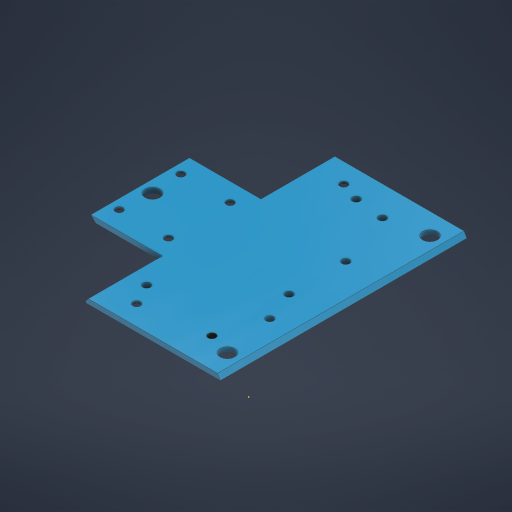
# Autodesk Inventor part: podstawa
Saved by Autodesk Inventor 2024 (Build 280153000, 153)
## iProperties
Created: 2024-05-21
Part Number: podstawa
Material: Steel
Document SubType Name: Modeling
Designer: Adam
Density: 7.85 g/cm^3
Appearance: Plate
Mass: 100.47 g
Surface Area: 136.936 cm^2
Volume: 12.7988 cm^3
Author: Adam
Autodesk Inventor part; units mm, degrees
ref_plane "YZ Plane" through (0, 0, 0) normal (1, 0, 0) x (0, 1, 0)
ref_plane "XZ Plane" through (0, 0, 0) normal (0, 1, 0) x (-1, 0, 0)
ref_plane "XY Plane" through (0, 0, 0) normal (0, 0, 1) x (1, 0, 0)
sketch "Sketch1" plane through (0, 0, 0) normal (0, 1, 0) x (-1, 0, 0)
  line L0 (0, 0) -> (0, -100)
  line L1 (0, -100) -> (66, -100)
  line L2 (66, -100) -> (66, -70)
  line L3 (66, -70) -> (94, -70)
  line L4 (94, -70) -> (94, -30)
  line L5 (94, -30) -> (66, -30)
  line L6 (66, -30) -> (66, 0)
  line L7 (66, 0) -> (0, 0)
  dimension "d0" = 100
  dimension "d2" = 30
  dimension "d4" = 40
  dimension "d7" = 66
  dimension "d27" = 94
  constraints: 16 end point, 4 perpendicular, 2 point on line, 1 parallel, 1 vertical
  measures "d0" distance of L0.start L0.end
  measures "d2" distance of L1.end L2.end
  measures "d4" distance of L3.end L4.end
  measures "d7" distance of L0.end L1.end
  measures "d27" distance between parallel lines of L0 L4
extrude "Extrusion1" add sketch "Sketch1" along normal blind 2
ref_plane "Work Plane1" through (-66, 0, -50) normal (0, 0, 1) x (1, 0, 0)
sketch "Sketch2" plane through (0, 0, 0) normal (0, -1, 0) x (1, 0, 0)
  point P0 (0, 0)
  point P1 (-69.9994, -37.5)
  point P2 (-90, -37.5)
  point P3 (-69.9994, -62.5)
  point P4 (-90, -62.5)
hole "Hole1" at (-90, 0, -37.5) at (-69.9994, 0, -37.5) at (-69.9994, 0, -62.5) at (-90, 0, -62.5) direction (0, 1, 0) diameter 3.1 end through all
chamfer "Chamfer1" distance 1.5 angle 45 4 edges at (-90, 0, -60.95) (-69.9994, 0, -60.95) (-69.9994, 0, -35.95) (-90, 0, -35.95) measured on face at (-69.9994, 0, -60.45) measured on face at (-90, 0, -60.45) measured on face at (-69.9994, 0, -35.45) measured on face at (-90, 0, -35.45)
chamfer "Chamfer2" distance 2 angle 45 1 edges at (-94, 0, -50)
sketch "Sketch3" plane through (-66, 0, -50) normal (0, 0, 1) x (1, 0, 0)
  line L0 (66, -6) -> (58, -6)
  line L1 (58, -6) -> (45.307, 15.985)
  line L2 (66, 0) -> (66, 2) projected
  line L3 (0, 0) -> (66, 0) projected
  line L4 (45.307, 15.985) -> (66, 15.985)
  line L5 (66, 15.985) -> (66, -6)
  line L6 (66, -6) -> (66, -6)
  point P0 (66, 1)
  dimension "d22" = 8
  dimension "d23" = 120
  dimension "d24" = 6
  constraints: 10 end point, 2 horizontal, 2 perpendicular, 2 point on line, 1 midpoint
  measures "d22" distance of L0.start L1.start
  measures "d23" angle of L0 L1
  measures "d24" distance between parallel lines of L3 L0
extrude "Extrusion2" cut sketch "Sketch3" along normal through all both and the other way through all
chamfer "Chamfer3" distance 1 distance2 1.2 2 edges at (-66, 2, -15) (-66, 2, -85) measured on face at (-65.5, 2, -85) measured on face at (-65.5, 2, -15)
sketch "Sketch4" plane through (0, 0, 0) normal (0, -1, 0) x (1, 0, 0)
  line L0 (-67.7565, -100) -> (-11.4641, -100)
  line L1 (-11.4641, -100) -> (-11.4641, 0)
  line L2 (-11.4641, 0) -> (-67.7565, 0)
  point P0 (0, 0)
  point P1 (-53.4039, -92)
  point P2 (-53.4039, -8)
  point P3 (-11.4641, 0)
  dimension "d31" = 8
  dimension "d32" = 41.9398
  dimension "d33" = 41.9398
  dimension "d34" = 8
  dimension "d35" = 100
  constraints: 6 end point, 2 perpendicular, 1 coincident
  measures "d31" distance from line of L2 point (-53.404, -8)
  measures "d32" distance from line of L1 point (-53.404, -8)
  measures "d33" distance from line of L1 point (-53.404, -92)
  measures "d34" distance from line of L0 point (-53.404, -92)
  measures "d35" distance between parallel lines of L0 L2
hole "Hole2" at (-53.4039, 0, -92) at (-53.4039, 0, -8) direction (0, 1, 0) diameter 3.1 end through all
chamfer "Chamfer4" distance 1.5 angle 45 2 edges at (-53.4039, 0, -90.45) (-53.4039, 0, -6.45) measured on face at (-53.4039, 0, -89.95) measured on face at (-53.4039, 0, -5.95)
sketch "Sketch6" plane through (0, 2, 0) normal (0, 1, 0) x (1, 0, 0)
  line L0 (-11.4641, 100) -> (-11.4641, 0) projected
  line L1 (-12.6188, 100) -> (-11.4641, 100) projected
  line L2 (-12.6188, 0) -> (-12.6188, 100) projected
  line L3 (-11.4641, 0) -> (-12.6188, 0) projected
  line L4 (-12.6188, 100) -> (-65, 100) projected
  line L5 (-65, 0) -> (-12.6188, 0) projected
  line L6 (-12.6715, 100) -> (-66, 100)
  line L7 (-11.4641, 100) -> (-11.4641, 39.7608)
  point P0 (-25.8771, 42.265)
  point P1 (-25.8771, 65.3)
  point P2 (-33.7057, 88)
  point P3 (-26.8923, 12)
  dimension "d56" = 34.7
  dimension "d57" = 42.265
  dimension "d83" = 21.0869
  dimension "d84" = 12
  dimension "d85" = 12
  dimension "d87" = 14.2735
  dimension "d88" = 14.413
  dimension "d89" = 14.413
  constraints: 4 end point
  measures "d56" distance from line of L4 point (-25.877, 65.3)
  measures "d57" distance from line of L5 point (-25.877, 42.265)
  measures "d83" distance from line of L2 point (-33.706, 88)
  measures "d84" distance from line of point (-33.706, 88) L4
  measures "d85" distance from line of point (-26.892, 12) L5
  measures "d87" distance from line of L2 point (-26.892, 12)
  measures "d88" distance from line of L0 point (-25.877, 65.3)
  measures "d89" distance from line of L0 point (-25.877, 42.265)
hole "Hole3" at (-33.7057, 2, -88) at (-25.8771, 2, -65.3) at (-25.8771, 2, -42.265) at (-26.8923, 2, -12) direction (0, -1, 0) diameter 3.1 end through all
sketch "Sketch7" plane through (0, 0, 0) normal (0, -1, 0) x (1, 0, 0)
  point P0 (0, 0)
sketch "Sketch8" plane through (0, 0, 0) normal (0, -1, 0) x (1, 0, 0)
  point P0 (0, 0)
  point P1 (-17.8084, -91.4246)
  point P2 (-17.8084, -9.1996)
  point P3 (-89, -50)
  point P4 (-17.8084, -9.1996)
  point P5 (-17.8084, -91.4246)
  point P6 (-89, -50)
  constraints: 3 coincident
hole "Hole4" at (-17.8084, 0, -9.1996) at (-17.8084, 0, -91.4246) at (-89, 0, -50) direction (0, 1, 0) diameter 6 end through all
sketch "Sketch10" plane through (0, 2, 0) normal (0, 1, 0) x (1, 0, 0)
  line L0 (-12.6188, 0) -> (-65, 0)
  line L1 (-65, 0) -> (-12.6188, 0) projected
  point P0 (0, 0)
  point P1 (-57.924, 16.544)
  point P2 (-57.924, 16.544)
  point P3 (-45.6312, 89.2874)
  point P4 (-21.1675, 29.7559)
  constraints: 2 end point
hole "Hole6" at (-21.1675, 2, -29.7559) at (-45.6312, 2, -89.2874) at (-57.924, 2, -16.544) direction (0, -1, 0) diameter 3.1 end through all
body "Solid1"
